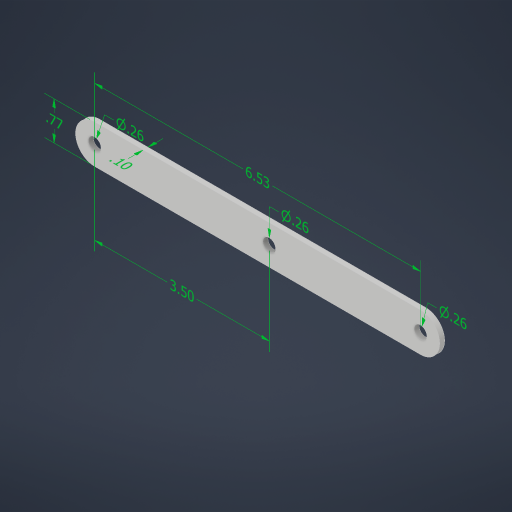
# Autodesk Inventor part: ArmConnector1Mini
Saved by Autodesk Inventor 2024.2 (Build 282272000, 272)
## iProperties
Created: 2019-01-19
Part Number: ArmConnector1Mini
Material: Generic
Document SubType Name: Modeling
Designer: Teacher
Density: 1 g/cm^3
Appearance: Default
Author: Teacher
Autodesk Inventor part; units mm, degrees
ref_plane "YZ Plane" through (0, 0, 0) normal (1, 0, 0) x (0, 1, 0)
ref_plane "XZ Plane" through (0, 0, 0) normal (0, 1, 0) x (-1, 0, 0)
ref_plane "XY Plane" through (0, 0, 0) normal (0, 0, 1) x (1, 0, 0)
sketch "Sketch1" plane through (0, 0, 0) normal (0, 0, 1) x (1, 0, 0)
  arc A0 (-94.4262, -10.1366) -> (-94.4262, 9.3452) centre (-94.4262, -0.3957) ccw
  arc A1 (-260.35, 9.3452) -> (-260.35, -10.1366) centre (-260.35, -0.3957) ccw
  line L0 (-260.35, 9.3452) -> (-94.4262, 9.3452)
  line L1 (-94.4262, -10.1366) -> (-260.35, -10.1366)
  circle A2 centre (-260.35, -0.3957) radius 3.2512
  circle A3 centre (-94.4262, -0.3957) radius 3.2512
  circle A4 centre (-171.45, -0.3957) radius 3.2512
  line L2 (-260.35, -0.3957) -> (-260.35, 9.3452) construction
  dimension "d0" = 19.4818
  dimension "d1" = 19.4818
  dimension "d3" = 6.5024
  dimension "d4" = 6.5024
  dimension "d12" = 6.5024
  dimension "d13" = 9.7409
  dimension "d14" = 88.9
  dimension "d19" = 90
  constraints: 6 end point, 5 centre point, 4 point on circle, 2 coincident, 2 tangent, 1 horizontal, 1 parallel, 1 vertical
  measures "d0" diameter of A0
  measures "d1" diameter of A1
  measures "d3" diameter of A2
  measures "d4" diameter of A3
  measures "d12" diameter of A4
  measures "d13" distance from line of L1 A4.centre
  measures "d14" distance of A1.centre A4.centre
  measures "d19" angle of L0 L2
extrude "Extrusion1" add sketch "Sketch1" along normal blind 2.54
equation "\"d0\" = d1"
body "Solid1"
